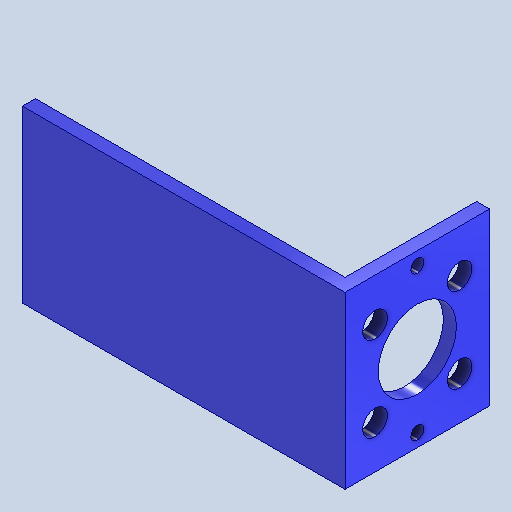
# Autodesk Inventor part: SoporteHidráhulicos_CPY
Saved by Autodesk Inventor 2023 (Build 270158000, 158)
## iProperties
Created: 2023-04-07
Part Number: SoporteHidráhulicos_CPY
Material: Steel, Mild, Welded
Document SubType Name: Modeling
Designer: Lenovo
Density: 7.85 g/cm^3
Appearance: Blue - Wall Paint - Glossy
Author: Lenovo
Autodesk Inventor part; units mm, degrees
ref_plane "YZ Plane" through (0, 0, 0) normal (1, 0, 0) x (0, 1, 0)
ref_plane "XZ Plane" through (0, 0, 0) normal (0, 1, 0) x (-1, 0, 0)
ref_plane "XY Plane" through (0, 0, 0) normal (0, 0, 1) x (1, 0, 0)
sketch "Sketch4" plane through (0, 0, 0) normal (1, 0, 0) x (0, 1, 0)
  line L0 (-6, -12.5) -> (-6, -12.9)
  arc A0 (-6, -12.9) -> (-5.6, -13.3) centre (-5.6, -12.9) ccw
  line L1 (-5.6, -13.3) -> (-4.9, -13.3)
  arc A1 (-4.9, -13.3) -> (-4.7, -13.1) centre (-4.9, -13.1) ccw
  line L2 (-4.7, -13.1) -> (-4.7, -12.85)
  arc A2 (-4.5, -12.65) -> (-4.7, -12.85) centre (-4.5, -12.85) ccw
  line L3 (-4.5, -12.65) -> (-1.8, -12.65)
  arc A3 (-1.4, -13.05) -> (-1.8, -12.65) centre (-1.8, -13.05) ccw
  line L4 (-1.4, -13.05) -> (-1.4, -18.75)
  line L5 (-1.8, -19.15) -> (-4.5, -19.15)
  arc A4 (-1.8, -19.15) -> (-1.4, -18.75) centre (-1.8, -18.75) ccw
  arc A5 (-4.7, -18.95) -> (-4.5, -19.15) centre (-4.5, -18.95) ccw
  line L6 (-4.7, -18.95) -> (-4.7, -18.7)
  arc A6 (-4.7, -18.7) -> (-4.9, -18.5) centre (-4.9, -18.7) ccw
  line L7 (-4.9, -18.5) -> (-5.6, -18.5)
  arc A7 (-5.6, -18.5) -> (-6, -18.9) centre (-5.6, -18.9) ccw
  line L8 (-6, -18.9) -> (-6, -19.5)
  line L9 (-6.5, -6.5) -> (-6.5, -12.5)
  line L10 (-6.5, -12.5) -> (-6, -12.5)
  line L11 (-6, -19.5) -> (-6.5, -19.5)
  line L12 (-6.5, -19.5) -> (-6.5, -26)
  line L13 (-6.5, -26) -> (-6, -26)
  line L14 (-6, -26) -> (-6, -26.6)
  arc A8 (-6, -26.6) -> (-5.6, -27) centre (-5.6, -26.6) ccw
  line L15 (-5.6, -27) -> (-4.9, -27)
  arc A9 (-4.9, -27) -> (-4.7, -26.8) centre (-4.9, -26.8) ccw
  arc A10 (-4.5, -26.35) -> (-4.7, -26.55) centre (-4.5, -26.55) ccw
  line L16 (-4.7, -26.8) -> (-4.7, -26.55)
  line L17 (-4.5, -26.35) -> (-1.8, -26.35)
  arc A11 (-1.4, -26.75) -> (-1.8, -26.35) centre (-1.8, -26.75) ccw
  line L18 (-1.4, -26.75) -> (-1.4, -32.45)
  arc A12 (-1.8, -32.85) -> (-1.4, -32.45) centre (-1.8, -32.45) ccw
  line L19 (-1.8, -32.85) -> (-4.5, -32.85)
  arc A13 (-4.7, -32.65) -> (-4.5, -32.85) centre (-4.5, -32.65) ccw
  line L20 (-4.7, -32.65) -> (-4.7, -32.4)
  arc A14 (-4.7, -32.4) -> (-4.9, -32.2) centre (-4.9, -32.4) ccw
  line L21 (-4.9, -32.2) -> (-5.6, -32.2)
  arc A15 (-5.6, -32.2) -> (-6, -32.6) centre (-5.6, -32.6) ccw
  line L22 (-6, -32.6) -> (-6, -33)
  line L23 (-6, -33) -> (-6.5, -33)
  line L24 (-6.5, -33) -> (-6.5, -39)
  circle A16 centre (0, -6.5) radius 4.75
  circle A17 centre (32.5, -6.5) radius 4.75
  circle A18 centre (0, -39) radius 4.75
  circle A19 centre (32.5, -39) radius 4.75
  line L25 (39, -26) -> (39, -19.5)
  line L26 (39, -12.5) -> (39, -6.5)
  line L27 (39, -39) -> (39, -33)
  line L28 (39, -45.5) -> (39, 0)
  line L29 (39, -45.5) -> (39, -55.5)
  line L30 (39, -55.5) -> (-6.5, -55.5)
  line L31 (-6.5, -55.5) -> (-6.5, -45.5)
  line L32 (39, 0) -> (39, 10)
  line L33 (39, 10) -> (-6.5, 10)
  line L34 (-6.5, 10) -> (-6.5, 0)
  line L35 (-6.5, 0) -> (-6.5, -12.5)
  line L36 (-6.5, -19.5) -> (-6.5, -26)
  line L37 (-6.5, -33) -> (-6.5, -45.5)
  line L38 (-6.5, 10) -> (-11.5, 10)
  line L39 (-11.5, 10) -> (-11.5, -55.5)
  line L40 (-11.5, -55.5) -> (-6.5, -55.5)
  line L41 (-6.5, -12.5) -> (-6.5, 10)
  line L42 (-6.5, -55.5) -> (-6.5, -33)
  line L43 (-6.5, -26) -> (-6.5, -19.5)
  point P0 (0, 0)
  dimension "d36" = 10
  dimension "d37" = 10
  dimension "d38" = 5
  constraints: 88 end point, 32 point on circle, 20 centre point, 9 parallel, 1 horizontal, 1 perpendicular, 1 point on line
  measures "d36" distance of L29.start L29.end
  measures "d37" distance of L32.end L32.start
  measures "d38" distance of L40.end L39.end
extrude "Extrusion6" add sketch "Sketch4" along normal blind 118.9 contours L0 A0 L1 A1 L2 A2 L3 A3 L4 A4 L5 A5 L6 A6 L7 A7 L8 L11 L12 L13 L14 A8 L15 A9 L16 A10 L17 A11 L18 A12 L19 A13 L20 A14 L21 A15 L22 L23 L24 L37 L31 L40 L39 L38 L34 L35 L9 L10
sketch "Sketch5" plane through (0, 0, 0) normal (-1, 0, 0) x (0, 0, 1)
  line L0 (-33, -6) -> (-32.6, -6)
  arc A0 (-32.6, -6) -> (-32.2, -5.6) centre (-32.6, -5.6) ccw
  line L1 (-32.2, -5.6) -> (-32.2, -4.9)
  arc A1 (-32.2, -4.9) -> (-32.4, -4.7) centre (-32.4, -4.9) ccw
  line L2 (-32.4, -4.7) -> (-32.65, -4.7)
  arc A2 (-32.85, -4.5) -> (-32.65, -4.7) centre (-32.65, -4.5) ccw
  line L3 (-32.85, -4.5) -> (-32.85, -1.8)
  arc A3 (-32.45, -1.4) -> (-32.85, -1.8) centre (-32.45, -1.8) ccw
  line L4 (-32.45, -1.4) -> (-26.75, -1.4)
  line L5 (-26.35, -1.8) -> (-26.35, -4.5)
  arc A4 (-26.35, -1.8) -> (-26.75, -1.4) centre (-26.75, -1.8) ccw
  arc A5 (-26.55, -4.7) -> (-26.35, -4.5) centre (-26.55, -4.5) ccw
  line L6 (-26.55, -4.7) -> (-26.8, -4.7)
  arc A6 (-26.8, -4.7) -> (-27, -4.9) centre (-26.8, -4.9) ccw
  line L7 (-27, -4.9) -> (-27, -5.6)
  arc A7 (-27, -5.6) -> (-26.6, -6) centre (-26.6, -5.6) ccw
  line L8 (-26.6, -6) -> (-26, -6)
  line L9 (-39, -6.5) -> (-33, -6.5)
  line L10 (-33, -6.5) -> (-33, -2.5)
  line L11 (-26, -1.05) -> (-26, -6.5)
  line L12 (-26, -6.5) -> (-19.5, -6.5)
  line L13 (-19.5, -6.5) -> (-19.5, -1.05)
  line L14 (-19.5, -6) -> (-18.9, -6)
  arc A8 (-18.9, -6) -> (-18.5, -5.6) centre (-18.9, -5.6) ccw
  line L15 (-18.5, -5.6) -> (-18.5, -4.9)
  arc A9 (-18.5, -4.9) -> (-18.7, -4.7) centre (-18.7, -4.9) ccw
  arc A10 (-19.15, -4.5) -> (-18.95, -4.7) centre (-18.95, -4.5) ccw
  line L16 (-18.7, -4.7) -> (-18.95, -4.7)
  line L17 (-19.15, -4.5) -> (-19.15, -1.8)
  arc A11 (-18.75, -1.4) -> (-19.15, -1.8) centre (-18.75, -1.8) ccw
  line L18 (-18.75, -1.4) -> (-13.05, -1.4)
  arc A12 (-12.65, -1.8) -> (-13.05, -1.4) centre (-13.05, -1.8) ccw
  line L19 (-12.65, -1.8) -> (-12.65, -4.5)
  arc A13 (-12.85, -4.7) -> (-12.65, -4.5) centre (-12.85, -4.5) ccw
  line L20 (-12.85, -4.7) -> (-13.1, -4.7)
  arc A14 (-13.1, -4.7) -> (-13.3, -4.9) centre (-13.1, -4.9) ccw
  line L21 (-13.3, -4.9) -> (-13.3, -5.6)
  arc A15 (-13.3, -5.6) -> (-12.9, -6) centre (-12.9, -5.6) ccw
  line L22 (-12.9, -6) -> (-12.5, -6)
  line L23 (-12.5, -2.5) -> (-12.5, -6.5)
  line L24 (-12.5, -6.5) -> (-6.5, -6.5)
  line L25 (-45.5, 32.5) -> (-45.5, 0)
  circle A16 centre (-39, 0) radius 4.75
  circle A17 centre (-39, 32.5) radius 4.75
  circle A18 centre (-6.5, 0) radius 4.75
  circle A19 centre (-6.5, 32.5) radius 4.75
  line L26 (-19.5, 39) -> (-26, 39)
  line L27 (-33, 39) -> (-39, 39)
  line L28 (-6.5, 39) -> (-12.5, 39)
  line L29 (0, 26.5) -> (0, 32.5)
  line L30 (0, 0) -> (0, 6)
  line L31 (0, 13) -> (0, 19.5)
  circle A20 centre (-22.75, 16.25) radius 15
  line L32 (-12.5, -6) -> (-12.5, -6.5) projected
  line L33 (10, -11.5) -> (-55.5, -11.5) projected
  line L34 (10, -11.5) -> (-55.5, -11.5)
  line L35 (-55.5, -11.5) -> (-55.5, 44)
  line L36 (-55.5, 44) -> (10, 44)
  line L37 (10, 44) -> (10, -11.5)
  line L38 (10, 39) -> (10, 44)
  point P0 (0, 0)
  point P1 (-55.5, -11.5)
  dimension "d43" = 5
  constraints: 74 end point, 32 point on circle, 21 centre point, 2 parallel, 1 collinear, 1 horizontal, 1 perpendicular, 1 vertical
  measures "d43" distance of L38.start L37.start
extrude "Extrusion7" add sketch "Sketch5" along normal blind 5
sketch "Sketch7" plane through (-5, 0, 0) normal (-1, 0, 0) x (0, 0, 1)
  line L0 (10, -11.5) -> (10, 44) projected
  line L1 (10, 44) -> (0, -11.5)
  line L2 (-55.5, -11.5) -> (10, -11.5) projected
  line L3 (10, -11.5) -> (0, 44)
  line L4 (10, 44) -> (-55.5, 44) projected
  line L5 (-55.5, 44) -> (-55.5, -11.5) projected
  line L6 (-55.5, -10.3017) -> (-45.7159, 44)
  line L7 (-45.7159, 44) -> (-55.5, 44)
  line L8 (-55.5, 44) -> (-45.5032, -11.4823)
  circle A0 centre (5, 16.25) radius 2.5
  circle A1 centre (-50.5016, 16.2588) radius 2.5
  point P0 (0, 0)
  dimension "d44" = 5
  dimension "d45" = 5
  constraints: 10 end point, 3 point on line, 2 centre point, 2 midpoint, 2 parallel, 1 horizontal
  measures "d44" diameter of A0
  measures "d45" diameter of A1
extrude "Extrusion8" cut sketch "Sketch7" against normal through all contours A0 L1 L3 | L3 L1 A0 | L1 L3 A0 | A0 L3 L1 | A1 L8 L6 | L6 L8 A1 | A1 L8 L6 | L6 L8 A1
body "Solid2"
